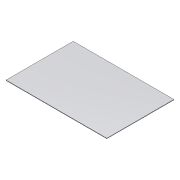
# Autodesk Inventor part: BellyPanConcept
Saved by Autodesk Inventor 2012 (Build 160160000, 160)
## iProperties
Created: 2013-01-08
Part Number: BellyPanConcept
Material: ABS Plastic
Document SubType Name: Modeling
Designer: JesseK
Density: 1.06 g/cm^3
Mass: 1328.83 g
Surface Area: 7983.85 cm^2
Volume: 1253.61 cm^3
Author: JesseK
Autodesk Inventor part; units mm, degrees
ref_plane "YZ Plane" through (0, 0, 0) normal (1, 0, 0) x (0, 1, 0)
ref_plane "XZ Plane" through (0, 0, 0) normal (0, 1, 0) x (-1, 0, 0)
ref_plane "XY Plane" through (0, 0, 0) normal (0, 0, 1) x (1, 0, 0)
sketch "Sketch2" plane through (0, 0, 0) normal (0, 1, 0) x (-1, 0, 0)
  line L0 (0, 0) -> (0, 457.2)
  line L1 (0, 457.2) -> (228.6, 457.2)
  line L2 (228.6, 457.2) -> (228.6, 457.2)
  line L3 (228.6, 457.2) -> (457.2, 457.2)
  line L4 (457.2, 457.2) -> (457.2, 457.2)
  line L5 (457.2, 457.2) -> (685.8, 457.2)
  line L6 (685.8, 457.2) -> (685.8, 0)
  line L7 (685.8, 0) -> (0, 0)
  dimension "d6" = 685.8
  dimension "d7" = 0
  dimension "d8" = 457.2
  dimension "d12" = 228.6
  constraints: 16 end point, 4 horizontal, 4 vertical, 2 collinear
  measures "d6" distance of L6.end L0.start
  measures "d7" distance between parallel lines of L3 L1
  measures "d8" distance between parallel lines of L7 L3
  measures "d12" distance of L0.end L1.end
extrude "Extrusion2" add sketch "Sketch2" along normal blind 3.175
body "Solid2"
